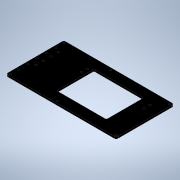
# Autodesk Inventor part: Sole
Saved by Autodesk Inventor 2020 (Build 240168000, 168)
## iProperties
Created: 2021-09-07
Part Number: Sole
Material: CFRP
Document SubType Name: Modeling
Designer: naoki
Density: 1.43 g/cm^3
Appearance: 黒
Author: naoki
Autodesk Inventor part; units mm, degrees
ref_plane "YZ Plane" through (0, 0, 0) normal (1, 0, 0) x (0, 1, 0)
ref_plane "XZ Plane" through (0, 0, 0) normal (0, 1, 0) x (-1, 0, 0)
ref_plane "XY Plane" through (0, 0, 0) normal (0, 0, 1) x (1, 0, 0)
sketch "スケッチ1" plane through (0, 0, 0) normal (0, 1, 0) x (-1, 0, 0)
  line L0 (-88.25, 46.25) -> (88.25, 46.25)
  line L1 (88.25, 46.25) -> (88.25, -46.25)
  line L2 (88.25, -46.25) -> (-88.25, -46.25)
  line L3 (-88.25, -46.25) -> (-88.25, 46.25)
  line L4 (-88.25, 46.25) -> (88.25, -46.25) construction
  line L5 (88.25, 46.25) -> (-88.25, -46.25) construction
  circle A0 centre (84.75, 42.75) radius 1.55
  circle A1 centre (9.75, 42.75) radius 1.55
  circle A2 centre (-84.75, 42.75) radius 1.55
  line L6 (151.0272, 0) -> (-157.6431, 0) construction
  line L7 (0, 129.3763) -> (0, -94.6315) construction
  circle A3 centre (84.75, -42.75) radius 1.55
  circle A4 centre (9.75, -42.75) radius 1.55
  circle A5 centre (-84.75, -42.75) radius 1.55
  circle A6 centre (30, -25.75) radius 1.55
  circle A7 centre (30, -16.25) radius 1.55
  line L8 (88.25, -25.75) -> (-88.25, -25.75) construction
  line L9 (-88.25, -16.25) -> (88.25, -16.25) construction
  circle A8 centre (-70.5, -25.75) radius 1.55
  circle A9 centre (-70.5, -16.25) radius 1.55
  circle A10 centre (84.75, -29.75) radius 1.55
  circle A11 centre (84.75, -14.75) radius 1.55
  circle A12 centre (84.75, 0.25) radius 1.55
  circle A13 centre (84.75, 15.25) radius 1.55
  circle A14 centre (84.75, 30.25) radius 1.55
  circle A15 centre (76.5, -25.75) radius 1.55
  circle A16 centre (76.5, -13.75) radius 1.55
  circle A17 centre (76.5, -1.75) radius 1.55
  circle A18 centre (76.5, 10.25) radius 1.55
  line L10 (-55.5, -30.75) -> (24.5, -30.75)
  line L11 (24.5, -30.75) -> (24.5, 29.25)
  line L12 (24.5, 29.25) -> (-55.5, 29.25)
  line L13 (-55.5, 29.25) -> (-55.5, -30.75)
  line L14 (-55.5, -30.75) -> (24.5, 29.25) construction
  line L15 (24.5, -30.75) -> (-55.5, 29.25) construction
  point P0 (0, 0)
  point P1 (-15.5, -0.75)
  dimension "d105" = 176.5
  dimension "d106" = 92.5
  dimension "d107" = 3.5
  dimension "d108" = 3.5
  dimension "d109" = 3.1
  dimension "d110" = 78.5
  dimension "d111" = 3.5
  dimension "d112" = 3.1
  dimension "d113" = 173
  dimension "d114" = 3.5
  dimension "d115" = 3.1
  dimension "d116" = 46.25
  dimension "d117" = 88.25
  dimension "d118" = 58.25
  dimension "d119" = 20.5
  dimension "d120" = 30
  dimension "d121" = 3.1
  dimension "d122" = 3.1
  dimension "d123" = 58.25
  dimension "d129" = 3.1
  dimension "d130" = 3.1
  dimension "d132" = 9.5
  dimension "d133" = 20.5
  dimension "d134" = 30
  dimension "d135" = 158.75
  dimension "d136" = 16.5
  dimension "d137" = 3.5
  dimension "d138" = 3.1
  dimension "d141" = 15
  dimension "d146" = 20.5
  dimension "d147" = 11.75
  dimension "d148" = 3.1
  dimension "d151" = 12
  dimension "d156" = 15.5
  dimension "d157" = 75.5
  dimension "d158" = 63.75
  dimension "d159" = 143.75
  dimension "d164" = 100.5
  constraints: 32 end point, 19 centre point, 6 point on line, 5 perpendicular, 4 midpoint, 4 parallel, 3 horizontal, 3 symmetric about line, 3 vertical, 17 other
  measures "d105" distance of L1.end L2.end
  measures "d106" distance of L0.end L1.end
  measures "d107" distance from line of L1 A0.centre
  measures "d108" distance from line of L0 A0.centre
  measures "d109" diameter of A0
  measures "d110" distance from line of L1 A1.centre
  measures "d111" distance from line of L0 A1.centre
  measures "d112" diameter of A1
  measures "d113" distance from line of A2.centre L1
  measures "d114" distance from line of L0 A2.centre
  measures "d115" diameter of A2
  measures "d116" distance between parallel lines of L0 L6
  measures "d117" distance between parallel lines of L1 L7
  measures "d118" distance from line of L1 A6.centre
  measures "d119" distance from line of L2 A6.centre
  measures "d120" distance from line of L2 A7.centre
  measures "d121" diameter of A6
  measures "d122" diameter of A7
  measures "d123" distance from line of L1 A7.centre
  measures "d129" diameter of A8
  measures "d130" diameter of A9
  measures "d132" distance of A8.centre A9.centre
  measures "d133" distance from line of L2 A8.centre
  measures "d134" distance from line of L2 A9.centre
  measures "d135" distance from line of L1 A9.centre
  measures "d136" distance from line of L2 A10.centre
  measures "d137" distance from line of L1 A10.centre
  measures "d138" diameter of A10
  measures "d141" distance of A10.centre A11.centre
  measures "d146" distance from line of L2 A15.centre
  measures "d147" distance of L8.start A15.centre
  measures "d148" diameter of A15
  measures "d151" distance of A15.centre A16.centre
  measures "d156" distance between parallel lines of L2 L10
  measures "d157" distance between parallel lines of L2 L12
  measures "d158" distance between parallel lines of L1 L11
  measures "d159" distance between parallel lines of L1 L13
  measures "d164" distance of A8.centre A6.centre
extrude "押し出し1" add sketch "スケッチ1" along normal blind 3
fillet "フィレット1" radius 2 4 edges at (-24.5, 1.5, 29.25) (-24.5, 1.5, -30.75) (55.5, 1.5, 29.25) (55.5, 1.5, -30.75)
fillet "フィレット2" radius 3 4 edges at (-88.25, 1.5, 46.25) (-88.25, 1.5, -46.25) (88.25, 1.5, 46.25) (88.25, 1.5, -46.25)
equation "\"d108\" = d107"
equation "\"d111\" = d107"
equation "\"d112\" = d109"
equation "\"d114\" = d111"
equation "\"d115\" = d112"
equation "\"d121\" = d109"
equation "\"d122\" = d109"
equation "\"d123\" = d118"
equation "\"d129\" = d131"
equation "\"d130\" = d131"
equation "\"d135\" = d128"
equation "\"d138\" = d109"
equation "\"d148\" = d138"
equation "\"d131\" = 3.1"
equation "\"d128\" = 158.75"
